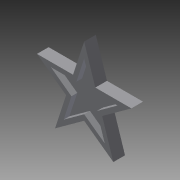
# Autodesk Inventor part: star
Saved by Autodesk Inventor 2015 SP1 (Build 190203100, 203)
## iProperties
Created: 2014-10-15
Part Number: star
Material: Generic
Document SubType Name: Modeling
Designer: dorislee
Density: 1 g/cm^3
Appearance: Default
Author: dorislee
Autodesk Inventor part; units mm, degrees
ref_plane "YZ Plane" through (0, 0, 0) normal (1, 0, 0) x (0, 1, 0)
ref_plane "XZ Plane" through (0, 0, 0) normal (0, 1, 0) x (-1, 0, 0)
ref_plane "XY Plane" through (0, 0, 0) normal (0, 0, 1) x (1, 0, 0)
sketch "Sketch1" plane through (0, 0, 0) normal (0, 0, 1) x (1, 0, 0)
  line L0 (13.5887, 9.0357) -> (17.6464, 0.3338)
  line L1 (17.6464, 0.3338) -> (27.6408, 0)
  line L2 (27.6408, 0) -> (21.4723, -7.8708)
  line L3 (21.4723, -7.8708) -> (25.567, -16.652)
  line L4 (25.567, -16.652) -> (13.4202, -12.2614)
  line L5 (13.5887, 2.702) -> (13.5887, 2.6795)
  line L6 (13.5887, 9.0357) -> (9.5309, 0.3338)
  line L7 (9.5309, 0.3338) -> (-0.4635, 0)
  line L8 (-0.4635, 0) -> (5.7051, -7.8708)
  line L9 (5.7051, -7.8708) -> (1.6103, -16.652)
  line L10 (1.6103, -16.652) -> (13.4202, -12.2614)
  line L11 (13.5887, 13) -> (8.102, 2.4963)
  line L12 (8.102, 2.4963) -> (-4.8863, 2.0624)
  line L13 (-4.8863, 2.0624) -> (3.1301, -8.1661)
  line L14 (3.1301, -8.1661) -> (-2.57, -20.39)
  line L15 (-2.57, -20.39) -> (13.3871, -14.6221)
  line L16 (13.5887, 13) -> (19.0899, 2.5183)
  line L17 (19.0899, 2.5183) -> (32.1087, 2.0834)
  line L18 (32.1087, 2.0834) -> (24.0735, -8.1691)
  line L19 (24.0735, -8.1691) -> (29.8589, -20.576)
  line L20 (29.8589, -20.576) -> (13.3871, -14.6221)
  point P0 (0, 0)
  dimension "d5" = 10
  dimension "d6" = 10
  constraints: 42 end point, 6 point on line, 4 symmetric about line, 1 vertical, 4 other
  measures "d5" distance of L0.end L1.end
  measures "d6" distance of L1.end L2.end
extrude "Extrusion1" [suppressed]
sketch "Sketch2" plane through (0, 0, 0) normal (0, 1, 0) x (-1, 0, 0)
  line L0 (0, 8.5065) -> (8.0902, 2.6287)
  line L1 (8.0902, 2.6287) -> (5, -6.8819)
  line L2 (5, -6.8819) -> (-5, -6.8819)
  line L3 (-5, -6.8819) -> (-8.0902, 2.6287)
  line L4 (-8.0902, 2.6287) -> (0, 8.5065)
  line L5 (0, 0) -> (0, 8.5065) construction
  line L6 (-5, -6.8819) -> (0, 8.5065)
  line L7 (5, -6.8819) -> (0, 8.5065)
  line L8 (-8.0902, 2.6287) -> (5, -6.8819)
  line L9 (-5, -6.8819) -> (8.0902, 2.6287)
  line L10 (8.0902, 2.6287) -> (-8.0902, 2.6287)
  point P0 (1.9098, 2.6287)
  point P1 (-1.9098, 2.6287)
  point P2 (-3.0902, -1.0041)
  point P3 (0, -3.2492)
  point P4 (3.0902, -1.0041)
  dimension "d13" = 10
  constraints: 22 end point, 10 point on line, 6 coincident, 1 horizontal, 1 vertical, 11 other
  measures "d13" distance of L0.start L0.end
extrude "Extrusion2" add sketch "Sketch2" along normal blind 2 contours L7 L10 L6 | L9 L7 L10 | L10 L6 L8 | L10 L7 L9 L8 L6 | L8 L9 L7 | L6 L8 L9
sketch "Sketch3" plane through (0, 0, 0) normal (0, -1, 0) x (1, 0, 0)
  line L0 (-5, -6.8819) -> (-3.0902, -1.0041) projected
  line L1 (0, -3.2492) -> (-5, -6.8819) projected
  line L2 (5, -6.8819) -> (0, -3.2492) projected
  line L3 (3.0902, -1.0041) -> (5, -6.8819) projected
  line L4 (8.0902, 2.6287) -> (3.0902, -1.0041) projected
  line L5 (1.9098, 2.6287) -> (8.0902, 2.6287) projected
  line L6 (0, 8.5065) -> (1.9098, 2.6287) projected
  line L7 (-1.9098, 2.6287) -> (0, 8.5065) projected
  line L8 (-8.0902, 2.6287) -> (-1.9098, 2.6287) projected
  line L9 (-3.0902, -1.0041) -> (-8.0902, 2.6287) projected
  line L10 (0, 6) -> (1.3471, 1.8541)
  line L11 (1.3471, 1.8541) -> (5.7063, 1.8541)
  line L12 (5.7063, 1.8541) -> (2.1796, -0.7082)
  line L13 (2.1796, -0.7082) -> (3.5267, -4.8541)
  line L14 (3.5267, -4.8541) -> (0, -2.2918)
  line L15 (0, -2.2918) -> (-3.5267, -4.8541)
  line L16 (-3.5267, -4.8541) -> (-2.1796, -0.7082)
  line L17 (-2.1796, -0.7082) -> (-5.7063, 1.8541)
  line L18 (-5.7063, 1.8541) -> (-1.3471, 1.8541)
  line L19 (-1.3471, 1.8541) -> (0, 6)
  point P0 (0, 0)
  dimension "d16" = 0.7745
  constraints: 20 end point, 9 other
  measures "d16" distance between parallel lines of L7 L19
extrude "Extrusion3" cut sketch "Sketch3" against normal blind 1 contours L10 L11 L12 L13 L14 L15 L16 L17 L18 L19
body "Solid1"
